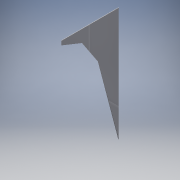
# Autodesk Inventor part: 15102898-16-P-0102
Saved by Autodesk Inventor 2017 (Build 210142000, 142)
## iProperties
Created: 2016-11-08
Part Number: 15102898-16-P-0102
Material: ABS Plastic
Document SubType Name: Modeling
Designer: gus
Density: 1.06 g/cm^3
Appearance: Smooth - Black
Author: gus
Autodesk Inventor part; units mm, degrees
ref_plane "YZ Plane" through (0, 0, 0) normal (1, 0, 0) x (0, 1, 0)
ref_plane "XZ Plane" through (0, 0, 0) normal (0, 1, 0) x (-1, 0, 0)
ref_plane "XY Plane" through (0, 0, 0) normal (0, 0, 1) x (1, 0, 0)
sketch "Sketch1" plane through (0, 0, 0) normal (1, 0, 0) x (0, 1, 0)
  line L0 (0, 0) -> (0, 355.6)
  line L1 (0, 355.6) -> (-50.8, 228.6)
  line L2 (-50.8, 228.6) -> (-203.2, 127)
  line L3 (-203.2, 127) -> (-685.8, 0)
  line L4 (-685.8, 0) -> (0, 0)
  dimension "d0" = 355.6
  dimension "d1" = 127
  dimension "d2" = 50.8
  dimension "d3" = 203.2
  dimension "d4" = 127
  dimension "d5" = 685.8
  constraints: 10 end point, 1 perpendicular, 1 vertical
  measures "d0" distance of L0.start L0.end
  measures "d1" vertical distance of L0.end L1.end
  measures "d2" distance from line of L0 L1.end
  measures "d3" distance from line of L0 L2.end
  measures "d4" distance from line of L2.end L4
  measures "d5" distance of L3.end L0.start
extrude "Extrusion1" add sketch "Sketch1" along normal blind 3.175
sketch "Sketch2" plane through (0, 0, 355.6) normal (0, 1, 0) x (1, 0, 0)
  line L0 (0, 355.6) -> (0, 0) projected
  line L1 (0, 0) -> (3.175, 0) projected
  line L2 (3.175, 355.6) -> (3.175, 0) projected
  line L3 (0, 355.6) -> (3.175, 355.6) projected
extrude "Extrusion2" add sketch "Sketch2" along normal blind 25.4
body "Solid1"
